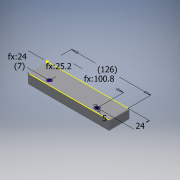
# Autodesk Inventor part: License_plate_mount
Saved by Autodesk Inventor 2019 (Build 230136000, 136)
## iProperties
Created: 2019-09-02
Part Number: License_plate_mount
Material: Generic
Document SubType Name: Modeling
Designer: steve
Density: 1 g/cm^3
Appearance: Default
Author: steve
Autodesk Inventor part; units mm, degrees
ref_plane "YZ Plane" through (0, 0, 0) normal (1, 0, 0) x (0, 1, 0)
ref_plane "XZ Plane" through (0, 0, 0) normal (0, 1, 0) x (-1, 0, 0)
ref_plane "XY Plane" through (0, 0, 0) normal (0, 0, 1) x (1, 0, 0)
sketch "Sketch1" plane through (0, 0, 0) normal (0, 0, 1) x (1, 0, 0)
  line L0 (2, 0) -> (128, 0)
  line L1 (130, 2) -> (130, 13)
  line L2 (128, 15) -> (2, 15)
  line L3 (0, 13) -> (0, 2)
  arc A0 (130, 13) -> (128, 15) centre (128, 13) ccw
  arc A1 (128, 0) -> (130, 2) centre (128, 2) ccw
  arc A2 (0, 2) -> (2, 0) centre (2, 2) ccw
  arc A3 (2, 15) -> (0, 13) centre (2, 13) ccw
  point P0 (0, 0)
  point P1 (130, 15)
  point P2 (130, 0)
  point P3 (0, 15)
  dimension "d0" = 130
  dimension "d1" = 15
  dimension "d2" = 2
  constraints: 8 end point, 8 point on circle, 8 point on line, 8 tangent, 4 centre point, 3 equal radius, 2 parallel, 1 horizontal, 1 perpendicular
  measures "d0" distance of point (130, 15) point (0, 15)
  measures "d1" distance of point (130, 0) point (130, 15)
  measures "d2" radius of A0
extrude "Extrusion1" add sketch "Sketch1" along normal blind 31
sketch "Sketch4" plane through (2, 15, 0) normal (0, 1, 0) x (1, 0, 0)
  circle A0 centre (100.8, -24) radius 2.5
  circle A1 centre (25.2, -24) radius 2.5
  line L0 (0, 0) -> (126, 0) projected
  line L1 (126, -31) -> (0, -31) projected
  point P0 (-2, 0)
  dimension "d31" = 5
  dimension "d32" = 100.8
  dimension "d33" = 126
  dimension "d34" = 25.2
  dimension "d35" = 24
  dimension "d36" = 24
  dimension "d42" = 7
  constraints: 2 centre point, 1 equal radius
  measures "d31" diameter of A0
  measures "d32" horizontal distance of L0.start A0.centre
  measures "d33" distance of L0.start L0.end
  measures "d34" horizontal distance of L0.start A1.centre
  measures "d35" distance from line of L0 A0.centre
  measures "d36" distance from line of L0 A1.centre
  measures "d42" distance from line of L1 A1.centre
extrude "Extrusion5" cut sketch "Sketch4" against normal up to next
sketch "Sketch5" plane through (2, 15, 0) normal (0, 1, 0) x (1, 0, 0)
  circle A0 centre (100.8, -24) radius 2.5 projected
  circle A1 centre (25.2, -24) radius 2.5 projected
  line L0 (98.4906, -20) -> (103.1094, -20)
  line L1 (103.1094, -20) -> (105.4188, -24)
  line L2 (105.4188, -24) -> (103.1094, -28)
  line L3 (103.1094, -28) -> (98.4906, -28)
  line L4 (98.4906, -28) -> (96.1812, -24)
  line L5 (96.1812, -24) -> (98.4906, -20)
  line L6 (22.8906, -20) -> (27.5094, -20)
  line L7 (27.5094, -20) -> (29.8188, -24)
  line L8 (29.8188, -24) -> (27.5094, -28)
  line L9 (27.5094, -28) -> (22.8906, -28)
  line L10 (22.8906, -28) -> (20.5812, -24)
  line L11 (20.5812, -24) -> (22.8906, -20)
  point P0 (-2, 0)
  point P1 (25.2, -28)
  point P2 (100.8, -28)
  dimension "d39" = 8
  constraints: 24 end point, 2 coincident, 2 horizontal, 2 midpoint, 1 equal length, 1 horizontal alignment, 26 other
  measures "d39" distance between parallel lines of L3 L0
extrude "Extrusion6" cut sketch "Sketch5" against normal blind 5 contours A1 | L0 L1 L2 L3 L4 L5 | L6 L7 L8 L9 L10 L11
equation "\"d32\" = 0.8 * d33"
equation "\"d34\" = 0.2 * d33"
equation "\"d36\" = d35"
body "Solid1"
